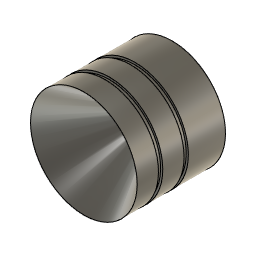
Nozzle (Autodesk Fusion 360 design; units mm, degrees)
Autodesk Fusion 360 part; units mm, degrees
sketch "Sketch1" plane through (0, 0, 0) normal (1, 0, 0) x (0, 1, 0)
  line L0 (0, 0) -> (0, 6.5)
  line L1 (0, 6.5) -> (13, 9.9833)
  line L2 (0, 6.5) -> (200, 6.5) construction
  line L3 (0, 0) -> (0, 6.5)
  line L4 (0, 10) -> (13, 10)
  line L5 (13, 10) -> (13, 6.5)
  line L6 (-2, 6.5) -> (0, 6.5)
  line L7 (-2, 0) -> (0, 0)
  line L8 (-2, 6.5) -> (-28.4207, 25)
  line L9 (-2, 6.5) -> (198, 6.5) construction
  line L10 (0, 25) -> (-28.4207, 25)
  line L11 (0, 0) -> (0, 6.5)
  line L12 (0, 10) -> (0, 25)
  line L13 (13, 9.9833) -> (13, 25)
  line L14 (13, 25) -> (0, 25)
  line L15 (-28.4207, 25) -> (-18.4207, 25)
  line L16 (-18.4207, 25) -> (-16.4207, 25)
  line L17 (-16.4207, 25) -> (-16.4207, 24)
  line L18 (-16.4207, 24) -> (-18.4207, 24)
  line L19 (-18.4207, 24) -> (-18.4207, 25)
  line L20 (-16.4207, 25) -> (-6.4207, 25)
  line L21 (-6.4207, 25) -> (-4.4207, 25)
  line L22 (-4.4207, 25) -> (-4.4207, 24)
  line L23 (-4.4207, 24) -> (-6.4207, 24)
  line L24 (-6.4207, 24) -> (-6.4207, 25)
  dimension "d7" = 6.5
  dimension "d8" = 15
  dimension "d10" = 10
  dimension "d11" = 6.5
  dimension "d12" = 145
  dimension "d14" = 25
  dimension "d15" = 10
  dimension "d16" = 2
  dimension "d17" = 1
  dimension "d18" = 10
  dimension "d19" = 2
  dimension "d20" = 1
  constraint coincident L0.start L3.start
  constraint vertical L0
  constraint horizontal L2
  constraint parallel L0 L3
  constraint perpendicular L3 L4
  constraint perpendicular L2 L5
  constraint perpendicular L0 L6
  constraint horizontal L9
  constraint perpendicular L7 L11
  constraint perpendicular L10 L11
  constraint coincident L2 L5.end
  constraint collinear L11 L12
  constraint coincident L5 L1.end
  constraint perpendicular L4 L13
  constraint parallel L10 L15
  constraint horizontal L16
  constraint vertical L17
  constraint horizontal L18
  constraint vertical L19
  constraint perpendicular L17 L20
  constraint horizontal L21
  constraint vertical L22
  constraint horizontal L23
  constraint vertical L24
  measures "d7" distance of L0.start L0.end
  measures "d8" angle of L1 L2
  measures "d10" distance of L0.start L4.start
  measures "d11" distance of L6.start L7.start
  measures "d12" angle of L8 L9
  measures "d14" distance of L0.start L10.start
  measures "d15" distance of L8.end L15.end
  measures "d16" distance of L15.end L16.end
  measures "d17" distance of L15.end L18.end
  measures "d18" distance of L16.end L20.end
  measures "d19" distance of L20.end L21.end
  measures "d20" distance of L20.end L23.end
revolve "Revolve1" add sketch "Sketch1" angle 360 about axis through (0, 1.75, 0) along (0, 1, 0) contours L1 L4 L5 L6 L8 L10 L12 L13 L15 L17 L18 L19 L20 L22 L23 L24 | L4 L12 L13 L14
